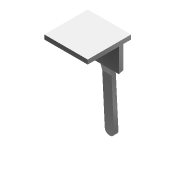
# Autodesk Inventor part: pin_2
Saved by Autodesk Inventor 2014 (Build 180170000, 170)
## iProperties
Created: 2015-10-12
Part Number: pin_2
Material: Generic
Document SubType Name: Modeling
Designer: Tom
Density: 1 g/cm^3
Appearance: Default
Author: Tom
Autodesk Inventor part; units mm, degrees
ref_plane "YZ Plane" through (0, 0, 0) normal (1, 0, 0) x (0, 1, 0)
ref_plane "XZ Plane" through (0, 0, 0) normal (0, 1, 0) x (-1, 0, 0)
ref_plane "XY Plane" through (0, 0, 0) normal (0, 0, 1) x (1, 0, 0)
sketch "Sketch1" plane through (0, 0, 0) normal (0, 0, 1) x (1, 0, 0)
  line L0 (0, 0) -> (2.413, 0)
  line L1 (2.413, 0) -> (2.413, 3.175)
  line L2 (2.413, 3.175) -> (0, 3.175)
  line L3 (0, 3.175) -> (0, 0)
  dimension "d0" = 2.413
  dimension "d1" = 3.175
  constraints: 8 end point, 2 parallel, 1 horizontal, 1 perpendicular
  measures "d0" distance of L2.end L1.end
  measures "d1" distance of L0.end L1.end
extrude "Extrusion1" add sketch "Sketch1" along normal blind 0.381
sketch "Sketch2" plane through (2.413, 0, 0) normal (1, 0, 0) x (0, 0, -1)
  line L0 (0, 3.175) -> (-0.381, 3.175) projected
  line L1 (0, 0) -> (-0.381, 0) projected
  line L2 (-0.381, 0) -> (-0.2241, -0.5857)
  line L3 (0, 0) -> (0.1569, -0.5857)
  line L4 (-0.2253, -0.5809) -> (0.0185, -5.461)
  line L5 (0.1562, -0.5831) -> (0.3999, -5.461)
  line L6 (-0.381, 0) -> (-0.381, 3.175) projected
  line L7 (0.0185, -5.461) -> (0.3999, -5.461)
  dimension "d5" = 0.381
  dimension "d6" = 8.636
  constraints: 10 end point, 2 parallel, 2 point on line, 1 perpendicular
  measures "d5" distance between parallel lines of L5 L4
  measures "d6" distance from line of L0 L4.end
extrude "Extrusion2" add sketch "Sketch2" against normal up to surface (2.413 mm away)
sketch "Sketch3" plane through (2.413, -5.461, -0.0185) normal (0, -0.0499, 0.9988) x (1, 0, 0)
  line L0 (-2.413, 4.8862) -> (-2.413, 0) projected
  line L1 (0, 4.8862) -> (-2.413, 4.8862) projected
  line L2 (-2.413, 5.4741) -> (0, 5.4741) projected
  line L3 (-2.413, -0.5509) -> (-1.6129, -0.5509)
  line L4 (-1.6129, -0.5509) -> (-1.6129, 4.8862)
  line L5 (-1.6129, 5.4741) -> (-2.413, 5.4741)
  line L6 (-2.413, 4.8862) -> (-2.413, -0.5509)
  line L7 (-0.4584, 5.4741) -> (0, 5.4741)
  line L8 (0, 5.4741) -> (0, 0)
  line L9 (-0.8001, -0.511) -> (0, -0.511)
  line L10 (-0.8001, -0.511) -> (-0.8001, 4.8862)
  line L11 (0, 4.8862) -> (0, -0.511)
  line L12 (-0.8001, 4.8862) -> (0, 4.8862)
  line L13 (-1.6129, 4.8862) -> (-2.413, 4.8862)
  point P0 (-2.413, 5.4551)
  dimension "d9" = 0.8128
  dimension "d10" = 2.413
  dimension "d11" = 0.8001
  constraints: 22 end point, 4 point on line, 3 parallel, 3 perpendicular, 2 collinear, 2 horizontal, 3 other
  measures "d9" horizontal distance of L3.end L9.start
  measures "d10" distance of L1.start L0.start
  measures "d11" distance of L9.start L9.end
extrude "Extrusion3" cut sketch "Sketch3" against normal through all
sketch "Sketch4" plane through (0, 0, 0.381) normal (0, -0.2588, 0.9659) x (1, 0, 0)
  line L0 (0, 0) -> (2.413, 0) projected
  line L1 (1.6129, -0.7023) -> (2.413, -0.7023)
  line L2 (2.413, -0.7023) -> (2.413, 0)
  line L3 (2.413, 0) -> (1.6129, 0)
  line L4 (1.6129, 0) -> (1.6129, -0.7023)
  line L5 (0, -0.7023) -> (0.8001, -0.7023)
  line L6 (0.8001, -0.7023) -> (0.8001, 0)
  line L7 (0.8001, 0) -> (0, 0)
  line L8 (0, 0) -> (0, -0.7023)
  point P0 (0, -0.0986)
  constraints: 16 end point, 4 parallel, 2 horizontal, 2 perpendicular, 1 point on line
extrude "Extrusion4" cut sketch "Sketch4" against normal through all
sketch "Sketch5" plane through (0, 3.175, 0) normal (0, 1, 0) x (1, 0, 0)
  line L0 (2.413, 0) -> (0, 0) projected
  line L1 (0, 0) -> (0, -0.381) projected
  line L2 (2.413, -0.381) -> (0, -0.381) projected
  line L3 (2.413, 0) -> (2.413, -0.381) projected
  line L4 (-0.6985, 0) -> (3.1115, 0)
  line L5 (3.1115, 0) -> (3.1115, -3.81)
  line L6 (3.1115, -3.81) -> (-0.6985, -3.81)
  line L7 (-0.6985, -3.81) -> (-0.6985, 0)
  dimension "d16" = 3.81
  dimension "d17" = 3.81
  dimension "d18" = 2.413
  dimension "d19" = 0.6985
  constraints: 8 end point, 2 parallel, 1 horizontal, 1 perpendicular
  measures "d16" distance of L5.end L6.end
  measures "d17" distance of L4.end L5.end
  measures "d18" distance of L2.start L1.end
  measures "d19" distance from line of L3 L4.end
extrude "Extrusion5" add sketch "Sketch5" against normal blind 0.381 contours L4 L5 L6 L7 L1 L2 L3
fillet "Fillet1" radius 0.381 2 edges at (0.8001, -5.461, -0.2092) (1.6129, -5.461, -0.2092)
equation "\"d11\" = -0.5 * d9 + 0.5 * d10"
equation "\"d19\" = -0.5 * d18 + 0.5 * d16"
body "Solid1"
